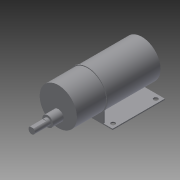
# Autodesk Inventor part: mfa_970d471
Saved by Autodesk Inventor 2014 SP1 (Build 180222100, 222)
## iProperties
Created: 2015-08-03
Part Number: mfa_970d471
Material: Générique
Document SubType Name: Modeling
Designer: astralien3000
Density: 1 g/cm^3
Appearance: Par défaut
Author: astralien3000
Autodesk Inventor part; units mm, degrees
ref_plane "YZ Plane" through (0, 0, 0) normal (1, 0, 0) x (0, 1, 0)
ref_plane "XZ Plane" through (0, 0, 0) normal (0, 1, 0) x (-1, 0, 0)
ref_plane "XY Plane" through (0, 0, 0) normal (0, 0, 1) x (1, 0, 0)
sketch "Esquisse1" plane through (0, 0, 0) normal (0, 1, 0) x (-1, 0, 0)
  circle A0 centre (0, 0) radius 18.25
  line L0 (-15, 0) -> (15, 0)
  line L1 (15, 0) -> (15, -20.05)
  line L2 (15, -20.05) -> (-15, -20.05)
  line L3 (-15, -20.05) -> (-15, 0)
  line L4 (-23.5, -21.05) -> (23.5, -21.05)
  line L5 (23.5, -21.05) -> (23.5, -20.05)
  line L6 (23.5, -20.05) -> (-23.5, -20.05)
  line L7 (-23.5, -20.05) -> (-23.5, -21.05)
  dimension "d0" = 36.5
  dimension "d1" = 30
  dimension "d2" = 15
  dimension "d3" = 1
  dimension "d4" = 47
  dimension "d5" = 23.5
  dimension "d6" = 39.3
  constraints: 16 end point, 4 parallel, 2 horizontal, 2 perpendicular, 1 centre point, 1 coincident, 1 collinear, 1 midpoint
  measures "d0" diameter of A0
  measures "d1" distance between parallel lines of L3 L1
  measures "d2" distance from line of L3 point (0, 0)
  measures "d3" distance between parallel lines of L4 L6
  measures "d4" distance of L4.start L4.end
  measures "d5" horizontal distance of point (0, 0) L5.end
extrude "Extrusion1" add sketch "Esquisse1" along normal blind 1
sketch "Esquisse2" plane through (0, 1, 0) normal (0, 1, 0) x (1, 0, 0)
  arc A0 (-15, 10.3953) -> (15, 10.3953) centre (0, 0) ccw projected
  circle A1 centre (0, 0) radius 17.5
  dimension "d9" = 35
  constraints: 1 centre point, 1 coincident
  measures "d9" diameter of A1
extrude "Extrusion2" add sketch "Esquisse2" along normal blind 50
sketch "Esquisse3" plane through (0, 0, 0) normal (0, -1, 0) x (1, 0, 0)
  arc A0 (15, -10.3953) -> (-15, -10.3953) centre (0, 0) ccw projected
  circle A1 centre (0, 0) radius 17.5
  dimension "d12" = 35
  constraints: 1 centre point, 1 coincident
  measures "d12" diameter of A1
extrude "Extrusion3" add sketch "Esquisse3" along normal blind 27.5
sketch "Esquisse4" plane through (0, 1, 0) normal (0, 1, 0) x (1, 0, 0)
  line L0 (-23.5, 21.05) -> (23.5, 21.05)
  line L1 (23.5, 21.05) -> (23.5, 20.05)
  line L2 (23.5, 20.05) -> (-23.5, 20.05)
  line L3 (-23.5, 20.05) -> (-23.5, 21.05)
  constraints: 8 end point, 2 parallel, 1 horizontal, 1 perpendicular
extrude "Extrusion4" add sketch "Esquisse4" along normal blind 48
sketch "Esquisse5" plane through (0, -27.5, 0) normal (0, -1, 0) x (1, 0, 0)
  circle A0 centre (0, 0) radius 17.5 projected
  line L0 (0, 0) -> (0, -17.5)
  circle A1 centre (0, -7) radius 5
  dimension "d17" = 7
  dimension "d18" = 10
  constraints: 2 end point, 1 centre point, 1 point on line, 1 vertical, 1 vertical alignment, 1 other
  measures "d17" distance of A1.centre L0.start
  measures "d18" diameter of A1
extrude "Extrusion5" add sketch "Esquisse5" along normal blind 10 contours A1 L0 | L0 A1
sketch "Esquisse6" plane through (0, -37.5, -7) normal (0, -1, 0) x (1, 0, 0)
  circle A0 centre (0, 0) radius 5 projected
  circle A1 centre (0, 0) radius 3
  point P0 (0, 7)
  dimension "d21" = 6
  constraints: 1 centre point, 1 coincident
  measures "d21" diameter of A1
extrude "Extrusion6" add sketch "Esquisse6" along normal blind 15 contours A1
sketch "Esquisse7" plane through (0, -52.5, -7) normal (0, -1, 0) x (1, 0, 0)
  circle A0 centre (0, 0) radius 3 projected
  line L0 (-1.6583, 2.5) -> (1.6583, 2.5)
  line L1 (1.6583, 2.5) -> (1.6583, 0)
  line L2 (1.6583, 0) -> (-1.6583, 0)
  line L3 (-1.6583, 0) -> (-1.6583, 2.5)
  arc A1 (1.6583, 2.5) -> (-1.6583, 2.5) centre (0, 0) ccw
  arc A2 (-1.6583, 2.5) -> (1.6583, 2.5) centre (0, 0) ccw
  point P0 (0, 7)
  dimension "d27" = 5.5
  constraints: 8 end point, 6 point on circle, 2 centre point, 2 parallel, 1 coincident, 1 concentric, 1 horizontal, 1 midpoint, 1 perpendicular
extrude "Extrusion7" cut sketch "Esquisse7" against normal blind 12 contours L0 A0
sketch "Esquisse8" plane through (0, 51, 0) normal (0, 1, 0) x (1, 0, 0)
  circle A0 centre (0, 0) radius 17.5 projected
  circle A1 centre (0, 0) radius 5
  dimension "d28" = 10
  constraints: 1 centre point, 1 coincident
  measures "d28" diameter of A1
extrude "Extrusion8" add sketch "Esquisse8" along normal blind 3 contours A1
sketch "Esquisse9" plane through (0, 54, 0) normal (0, 1, 0) x (1, 0, 0)
  circle A0 centre (0, 0) radius 5 projected
  circle A1 centre (0, 0) radius 1
  dimension "d31" = 2
  constraints: 1 centre point, 1 coincident
  measures "d31" diameter of A1
extrude "Extrusion9" add sketch "Esquisse9" along normal blind 3 contours A1
sketch "Esquisse10" plane through (23.5, 0, -21.05) normal (0, 0, -1) x (-1, 0, 0)
  line L0 (0, 0) -> (47, 0) projected
  line L1 (47, 0) -> (47, 49) projected
  line L2 (0, 49) -> (47, 49) projected
  line L3 (0, 0) -> (0, 49) projected
  line L4 (4, 44.5) -> (43, 44.5)
  line L5 (43, 44.5) -> (43, 4.5)
  line L6 (43, 4.5) -> (4, 4.5)
  line L7 (4, 4.5) -> (4, 44.5)
  point P0 (23.5, 0)
  dimension "d34" = 39
  dimension "d35" = 47
  dimension "d36" = 4
  dimension "d37" = 40
  dimension "d38" = 49
  dimension "d39" = 4.5
  constraints: 8 end point, 2 parallel, 1 horizontal, 1 perpendicular
  measures "d34" distance between parallel lines of L7 L5
  measures "d35" distance between parallel lines of L3 L1
  measures "d36" distance between parallel lines of L1 L5
  measures "d37" distance between parallel lines of L4 L6
  measures "d38" distance between parallel lines of L0 L2
  measures "d39" distance between parallel lines of L2 L4
hole "Perçage1" at (19.5, 44.5, -21.05) at (-19.5, 44.5, -21.05) at (-19.5, 4.5, -21.05) at (19.5, 4.5, -21.05) direction (0, 0, 1) diameter 4 end through all
equation "\"d2\" = 0.5 * d1"
equation "\"d5\" = 0.5 * d4"
equation "\"d36\" = -0.5 * d34 + 0.5 * d35"
equation "\"d39\" = -0.5 * d37 + 0.5 * d38"
